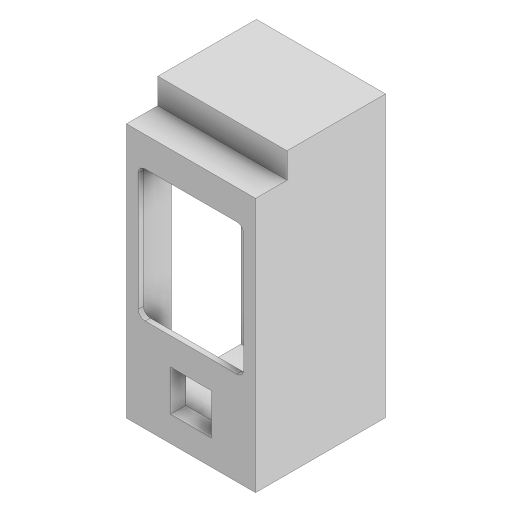
# Autodesk Inventor part: Part1
Saved by Autodesk Inventor 2023.3 (Build 273359000, 359)
## iProperties
Created: 2025-03-14
Part Number: Part1
Material: Generic
Document SubType Name: Modeling
Designer: David Zindović
Density: 1 g/cm^3
Appearance: Default
Author: David Zindović
Autodesk Inventor part; units mm, degrees
ref_plane "YZ Plane" through (0, 0, 0) normal (1, 0, 0) x (0, 1, 0)
ref_plane "XZ Plane" through (0, 0, 0) normal (0, 1, 0) x (-1, 0, 0)
ref_plane "XY Plane" through (0, 0, 0) normal (0, 0, 1) x (1, 0, 0)
sketch "Sketch1" plane through (0, 0, 0) normal (0, 0, 1) x (1, 0, 0)
  line L0 (-17, 22.5) -> (17, 22.5)
  line L1 (17, 22.5) -> (17, -22.5)
  line L2 (17, -22.5) -> (-17, -22.5)
  line L3 (-17, -22.5) -> (-17, 22.5)
  line L4 (-6, -25) -> (6, -25)
  line L5 (6, -25) -> (6, -37)
  line L6 (6, -37) -> (-6, -37)
  line L7 (-6, -37) -> (-6, -25)
  line L8 (-17, 28.5) -> (17, 28.5)
  line L9 (17, 28.5) -> (17, -29.5)
  line L10 (17, -29.5) -> (-17, -29.5)
  line L11 (-17, -29.5) -> (-17, 28.5)
  line L12 (-17, -29.5) -> (12, -29.5)
  line L13 (12, -29.5) -> (12, -42.5)
  line L14 (12, -42.5) -> (-17, -42.5)
  line L15 (-17, -42.5) -> (-17, -29.5)
  circle A0 centre (-14.5, -39.88) radius 1.5
  circle A1 centre (9.5, -39.88) radius 1.5
  circle A2 centre (-14.125, 25.5) radius 1.5
  circle A3 centre (14.125, 25.5) radius 1.5
  line L16 (-19, 30.5) -> (19, 30.5)
  line L17 (19, 30.5) -> (19, -44.5)
  line L18 (19, -44.5) -> (-19, -44.5)
  line L19 (-19, -44.5) -> (-19, 30.5)
  line L20 (12, -42.5) -> (17, -42.5)
  line L21 (17, -42.5) -> (17, -29.5)
  circle A4 centre (9.5, -39.88) radius 2.4
  circle A5 centre (-14.5, -39.88) radius 2.4
  circle A6 centre (14.125, 25.5) radius 2.4
  circle A7 centre (-14.125, 25.5) radius 2.4
  line L22 (-14.5, -36.7046) -> (-11.75, -38.2923)
  line L23 (-11.75, -38.2923) -> (-11.75, -41.4677)
  line L24 (-11.75, -41.4677) -> (-14.5, -43.0554)
  line L25 (-14.5, -43.0554) -> (-17.25, -41.4677)
  line L26 (-17.25, -41.4677) -> (-17.25, -38.2923)
  line L27 (-17.25, -38.2923) -> (-14.5, -36.7046)
  line L28 (-12.5373, 22.75) -> (-15.7127, 22.75)
  line L29 (-15.7127, 22.75) -> (-17.3004, 25.5)
  line L30 (-17.3004, 25.5) -> (-15.7127, 28.25)
  line L31 (-15.7127, 28.25) -> (-12.5373, 28.25)
  line L32 (-12.5373, 28.25) -> (-10.9496, 25.5)
  line L33 (-10.9496, 25.5) -> (-12.5373, 22.75)
  point P0 (0, 0)
  point P1 (0, 22.5)
  point P2 (17, 0)
  point P3 (0, -25)
  point P4 (0, -22.5)
  point P5 (0, 28.5)
  point P6 (-2.5, -42.5)
  point P7 (0, -44.5)
  point P8 (17, -22.5)
  dimension "d0" = 34
  dimension "d1" = 45
  dimension "d2" = 2.5
  dimension "d3" = 12
  dimension "d4" = 12
  dimension "d5" = 34
  dimension "d6" = 58
  dimension "d7" = 7
  dimension "d8" = 13
  dimension "d9" = 29
  dimension "d10" = 3
  dimension "d11" = 3
  dimension "d12" = 3
  dimension "d13" = 3
  dimension "d14" = 28.25
  dimension "d15" = 14.125
  dimension "d16" = 3
  dimension "d17" = 24
  dimension "d18" = 12
  dimension "d19" = 2.62
  dimension "d21" = 2
  dimension "d22" = 2
  dimension "d23" = 2
  dimension "d66" = 4.8
  dimension "d67" = 4.8
  dimension "d68" = 4.8
  dimension "d69" = 4.8
  dimension "d75" = 5.5
  dimension "d85" = 5.5
  constraints: 68 end point, 10 parallel, 8 centre point, 7 coincident, 7 midpoint, 6 horizontal, 5 perpendicular, 5 vertical alignment, 4 horizontal alignment, 1 collinear, 26 other
  measures "d0" distance of L0.start L0.end
  measures "d1" distance of L0.end L1.end
  measures "d2" distance between parallel lines of L2 L4
  measures "d3" distance of L5.end L6.end
  measures "d4" distance of L4.end L5.end
  measures "d5" distance of L8.start L8.end
  measures "d6" distance of L8.end L9.end
  measures "d7" distance between parallel lines of L2 L10
  measures "d8" distance of L12.end L13.end
  measures "d9" distance of L13.end L14.end
  measures "d10" diameter of A0
  measures "d11" diameter of A1
  measures "d12" diameter of A2
  measures "d13" diameter of A3
  measures "d14" distance of A3.centre A2.centre
  measures "d15" horizontal distance of point (0, 28.5) A3.centre
  measures "d16" distance from line of L8 A2.centre
  measures "d17" distance of A0.centre A1.centre
  measures "d18" horizontal distance of point (-2.5, -42.5) A1.centre
  measures "d19" distance from line of L14 A0.centre
  measures "d21" distance between parallel lines of L14 L18
  measures "d22" distance between parallel lines of L3 L19
  measures "d23" distance between parallel lines of L16 L8
  measures "d66" diameter of A4
  measures "d67" diameter of A5
  measures "d68" diameter of A6
  measures "d69" diameter of A7
  measures "d75" distance between parallel lines of L26 L23
  measures "d85" distance between parallel lines of L31 L28
extrude "Extrusion1" add sketch "Sketch1" along normal blind 4.5 contours L11 L29 L28 L33 L32 L31 L30 L8 L9 L0 | L2 L9 L10 L5 L4 L7 L11 | L29 L30 L11 | L11 L30 L31 L32 L33 L28 L29 | L10 L7 L6 L5 L13 L14 L24 L23 L22 L27 L15 | L21 L20 L13 L10 | L27 L22 L23 L24 L14 L25 L15 | L15 L25 L26 L27 | L25 L14 L15 | L14 L24 L25 | A0 | A1 | A2 | A3 | L16 L17 L18 L19 | A4 | A5 | A6 | A7
sketch "Sketch2" plane through (0, 0, 4.5) normal (0, 0, 1) x (1, 0, 0)
  line L0 (-17, -22.5) -> (-17, 22.5) projected
  line L1 (-17, 21.75) -> (17, 21.75)
  line L2 (17, 22.5) -> (17, -22.5) projected
  line L3 (-17, 22.5) -> (17, 22.5) projected
  line L4 (17, -22.5) -> (-17, -22.5) projected
  line L5 (-15.5, -22.5) -> (-15.5, 22.5)
  line L6 (-17, 22.5) -> (17, 22.5) projected
  line L7 (15.5, -22.5) -> (15.5, 22.5)
  line L8 (-17, -17) -> (17, -17)
  point P0 (0, 0)
  point P1 (-15.5, 21.75)
  point P2 (15.5, 21.75)
  point P3 (15.5, -17)
  point P4 (-15.5, -17)
  dimension "d26" = 0.75
  dimension "d27" = 1.5
  dimension "d28" = 1.5
  dimension "d29" = 5.5
  constraints: 8 end point, 8 point on line, 3 perpendicular, 1 horizontal
  measures "d26" distance between parallel lines of L3 L1
  measures "d27" distance between parallel lines of L0 L5
  measures "d28" distance between parallel lines of L2 L7
  measures "d29" distance between parallel lines of L8 L4
extrude "Extrusion2" add sketch "Sketch2" against normal blind 1.5 contours L0 L8 L5 L4 | L0 L1 L5 L8 | L5 L8 L7 L4 | L0 L3 L5 L1 | L7 L8 L2 L4 | L5 L3 L7 L1 | L7 L1 L2 L8 | L7 L3 L2 L1
fillet "Fillet1" radius 2 4 edges at (15.5, 21.75, 3.75) (-15.5, 21.75, 3.75) (-15.5, -17, 3.75) (15.5, -17, 3.75)
extrude "Extrusion3" add sketch "Sketch1" against normal blind 29.25 contours L29 L30 L11 | L15 L25 L26 L27 | L14 L24 L25 | L16 L17 L18 L19
sketch "Sketch3" plane through (-19, -44.5, 4.5) normal (-1, 0, 0) x (0, 0, 1)
  line L0 (-33.75, 2) -> (-33.75, 73) projected
  line L1 (-4.5, 2) -> (-33.75, 2) projected
  line L2 (-33.75, 73) -> (-11.25, 73)
  line L3 (-11.25, 73) -> (-11.25, 2)
  line L4 (-11.25, 2) -> (-33.75, 2)
  line L5 (-33.75, 2) -> (-33.75, 73)
  point P0 (-4.5, 44.5)
  dimension "d35" = 22.5
  constraints: 8 end point, 2 parallel, 1 horizontal, 1 perpendicular, 1 point on line
  measures "d35" distance of L3.end L4.end
extrude "Extrusion4" cut sketch "Sketch3" against normal up to surface (2 mm away)
sketch "Sketch4" plane through (0, 0, -29.25) normal (0, 0, -1) x (-1, 0, 0)
  line L0 (-19, 30.5) -> (-19, -44.5) projected
  line L1 (19, 30.5) -> (-19, 30.5) projected
  line L2 (-19, 30.5) -> (19, 30.5) projected
  line L3 (-19, 30.5) -> (19, 30.5)
  line L4 (19, 30.5) -> (19, -44.5)
  line L5 (19, -44.5) -> (-19, -44.5)
  line L6 (-19, -44.5) -> (-19, 30.5)
  point P0 (0, 0)
  constraints: 8 end point, 2 parallel, 1 horizontal, 1 perpendicular
extrude "Extrusion5" add sketch "Sketch4" along normal blind 2
sketch "Sketch5" plane through (-19, -44.5, 4.5) normal (-1, 0, 0) x (0, 0, 1)
  line L0 (-33.75, 73) -> (-11.25, 73) projected
  line L1 (-33.75, 73) -> (-11.25, 73)
  line L2 (-11.25, 73) -> (-11.25, 80.5)
  line L3 (-11.25, 80.5) -> (-33.75, 80.5)
  line L4 (-33.75, 80.5) -> (-33.75, 73)
  point P0 (-4.5, 44.5)
  dimension "d40" = 7.5
  constraints: 8 end point, 2 parallel, 1 horizontal, 1 perpendicular
  measures "d40" distance of L3.end L0.start
extrude "Extrusion6" cut sketch "Sketch5" against normal up to surface (36 mm away)
sketch "Sketch6" plane through (-19, -44.5, 4.5) normal (-1, 0, 0) x (0, 0, 1)
  line L0 (-33.75, 80.5) -> (-33.75, 73) projected
  line L1 (-11.25, 80.5) -> (-33.75, 80.5) projected
  line L2 (-11.25, 73) -> (-11.25, 80.5) projected
  line L3 (-35.75, 73) -> (-35.75, 82.5)
  line L4 (-35.75, 82.5) -> (-9.25, 82.5)
  line L5 (-9.25, 82.5) -> (-9.25, 73)
  line L6 (-35.75, 73) -> (-9.25, 73)
  line L7 (-4.5, 73) -> (-4.5, 67) projected
  point P0 (-4.5, 44.5)
  dimension "d43" = 2
  constraints: 8 end point, 1 perpendicular, 2 other
  measures "d43" distance between parallel lines of L1 L4
extrude "Extrusion7" add sketch "Sketch6" against normal up to surface (38 mm away) contours L0 L6 L3 L4 L5 L2 L1
sketch "Sketch7" plane through (19, -44.5, 4.5) normal (1, 0, 0) x (0, 0, -1)
  line L0 (11.25, 80.5) -> (11.25, 75) projected
  line L1 (33.75, 75) -> (11.25, 75) projected
  line L2 (33.75, 80.5) -> (11.25, 80.5) projected
  line L3 (33.75, 75) -> (33.75, 80.5) projected
  point P0 (4.5, 44.5)
extrude "Extrusion8" add sketch "Sketch7" against normal up to surface (2 mm away)
sketch "Sketch8" plane through (-17, -42.5, 0) normal (0, 1, 0) x (1, 0, 0)
  line L0 (34, 0) -> (34, 29.25) projected
  line L1 (-2, 29.25) -> (34, 29.25) projected
  line L2 (31.85, 29.25) -> (28.25, 29.25)
  line L3 (28.25, 29.25) -> (28.25, 20)
  line L4 (28.25, 20) -> (31.85, 20)
  line L5 (31.85, 20) -> (31.85, 29.25)
  point P0 (17, 0)
  dimension "d48" = 2.15
  dimension "d49" = 3.6
  dimension "d50" = 9.25
  constraints: 8 end point, 2 parallel, 1 horizontal, 1 perpendicular, 1 point on line
  measures "d48" distance between parallel lines of L0 L5
  measures "d49" distance of L3.end L4.end
  measures "d50" distance of L4.end L2.start
extrude "Extrusion9" cut sketch "Sketch8" against normal up to surface (2 mm away)
fillet "Fillet2" radius 0.75 4 edges at (14.85, -43.5, -29.25) (11.25, -43.5, -29.25) (11.25, -43.5, -20) (14.85, -43.5, -20)
sketch "Sketch9" plane through (17, -22.5, 3) normal (-1, 0, 0) x (0, 0, 1)
  circle A0 centre (-21.6, 19.25) radius 2.4
  line L0 (-9.75, -20) -> (-32.25, -20) projected
  line L1 (-32.25, -20) -> (-32.25, 58.5) projected
  circle A1 centre (-21.6, 19.25) radius 3.4
  point P0 (-3, 22.5)
  dimension "d54" = 4.8
  dimension "d55" = 39.25
  dimension "d56" = 10.65
  dimension "d57" = 1
  constraints: 2 centre point
  measures "d54" diameter of A0
  measures "d55" distance from line of L0 A0.centre
  measures "d56" distance from line of L1 A0.centre
  measures "d57" radial gap between concentric circles of A0 A1
extrude "Extrusion10" add sketch "Sketch9" along normal blind 3
chamfer "Chamfer1" distance 2 angle 45 1 edges at (17, -3.25, -22)
sketch "Sketch10" plane through (0, 0, -31.25) normal (0, 0, -1) x (-1, 0, 0)
  line L0 (12.6336, -38.0136) -> (16.3664, -38.0136) construction
  line L1 (16.3664, -38.0136) -> (16.3664, -41.7464) construction
  line L2 (16.3664, -41.7464) -> (12.6336, -41.7464) construction
  line L3 (12.6336, -41.7464) -> (12.6336, -38.0136) construction
  circle A0 centre (14.5, -39.88) radius 1.6
  circle A1 centre (14.125, 25.5) radius 1.6
  point P0 (0, 0)
  point P1 (14.5, -38.0136)
  point P2 (16.3664, -39.88)
  dimension "d64" = 3.7328
  dimension "d65" = 3.7328
  dimension "d95" = 3.2
  dimension "d96" = 3.2
  constraints: 8 end point, 2 centre point, 2 coincident, 2 midpoint, 2 parallel, 1 horizontal, 1 horizontal alignment, 1 perpendicular, 1 vertical alignment
  measures "d64" distance of L1.end L2.end
  measures "d65" distance of L0.end L1.end
  measures "d95" diameter of A0
  measures "d96" diameter of A1
extrude "Extrusion11" [suppressed]
sketch "Sketch11" plane through (-19, -44.5, 4.5) normal (0, -1, 0) x (1, 0, 0)
  line L0 (1.6, -3.7) -> (7.4, -3.7)
  line L1 (7.4, -3.7) -> (7.4, -1)
  line L2 (7.4, -1) -> (1.6, -1)
  line L3 (1.6, -1) -> (1.6, -3.7)
  line L4 (0, 0) -> (38, 0) projected
  point P0 (19, -4.5)
  point P1 (4.5, -4.5)
  point P2 (4.5, -3.7)
  dimension "d72" = 5.8
  dimension "d73" = 2.7
  dimension "d74" = 1
  constraints: 8 end point, 2 parallel, 1 horizontal, 1 midpoint, 1 perpendicular, 1 vertical alignment
  measures "d72" distance of L1.end L2.end
  measures "d73" distance of L2.end L0.start
  measures "d74" distance between parallel lines of L4 L2
extrude "Extrusion12" cut sketch "Sketch11" against normal up to surface (7.7954 mm away)
sketch "Sketch14" plane through (-19, -44.5, 4.5) normal (-1, 0, 0) x (0, 0, 1)
  line L0 (-3.7, 67.1) -> (-1, 67.1)
  line L1 (-1, 67.1) -> (-1, 72.9)
  line L2 (-1, 72.9) -> (-3.7, 72.9)
  line L3 (-3.7, 72.9) -> (-3.7, 67.1)
  line L4 (0, 75) -> (0, 0) projected
  point P0 (-4.5, 44.5)
  point P1 (-4.5, 70)
  point P2 (-3.7, 70)
  dimension "d86" = 5.8
  dimension "d87" = 2.7
  dimension "d88" = 1
  constraints: 8 end point, 2 parallel, 1 horizontal, 1 horizontal alignment, 1 midpoint, 1 perpendicular
  measures "d86" distance of L0.end L1.end
  measures "d87" distance of L0.start L0.end
  measures "d88" distance between parallel lines of L4 L1
extrude "Extrusion14" cut sketch "Sketch14" against normal up to surface (8.0504 mm away)
sketch "Sketch12" plane through (-11.6, -44.5, 3.5) normal (0, 0, -1) x (-1, 0, 0)
  line L0 (0, 0) -> (0, 7.7954) projected
  line L1 (5.8, 7.7954) -> (0, 7.7954) projected
  line L2 (5.8, 7.7954) -> (0, 7.7954) projected
  line L3 (0, 0) -> (0, 7.7954) projected
  line L4 (5.8, 0) -> (0, 0) projected
  line L5 (5.8, 0) -> (5.8, 7.7954) projected
  line L6 (2.9, 7.7954) -> (5.8, 6.1211)
  line L7 (5.65, 6.2077) -> (5.65, 3.0323)
  line L8 (5.65, 3.0323) -> (2.9, 1.4446)
  line L9 (2.9, 1.4446) -> (0.15, 3.0323)
  line L10 (0.15, 3.0323) -> (0.15, 6.2077)
  line L11 (0, 6.1211) -> (2.9, 7.7954)
  point P0 (-11.6, 44.5)
  point P1 (2.9, 4.62)
  dimension "d78" = 5.5
  constraints: 12 end point, 4 point on line, 2 midpoint, 2 vertical alignment, 13 other
  measures "d78" distance between parallel lines of L7 L10
extrude "Extrusion13" add sketch "Sketch12" along normal up to surface (2.7 mm away) contours L0 L1 L11 | L6 L1 L5
sketch "Sketch13" plane through (-19, 30.5, 4.5) normal (0, 1, 0) x (1, 0, 0)
  line L0 (7.775, 3.7) -> (1.975, 3.7)
  line L1 (1.975, 3.7) -> (1.975, 1)
  line L2 (1.975, 1) -> (7.775, 1)
  line L3 (7.775, 1) -> (7.775, 3.7)
  line L4 (38, 0) -> (0, 0) projected
  point P0 (19, 4.5)
  point P1 (7.775, 2.35)
  point P2 (1.975, 2.35)
  point P3 (4.875, 4.5)
  point P4 (4.875, 1)
  dimension "d81" = 5.8
  dimension "d82" = 2.7
  dimension "d83" = 1
  constraints: 8 end point, 3 midpoint, 2 parallel, 1 horizontal, 1 perpendicular, 1 vertical alignment
  measures "d81" distance of point (7.775, 2.35) point (1.975, 2.35)
  measures "d82" distance between parallel lines of L0 L2
  measures "d83" distance between parallel lines of L4 L2
sketch "Sketch15" plane through (-19, 22.6, 3.5) normal (0, 0, -1) x (-1, 0, 0)
  line L0 (-8.0504, 5.8) -> (-8.0504, 0) projected
  line L1 (0, 0) -> (-8.0504, 0) projected
  line L2 (0, 5.8) -> (0, 0) projected
  line L3 (0, 5.8) -> (-8.0504, 5.8) projected
  line L4 (-8.0504, 2.9) -> (-6.3761, 5.8)
  line L5 (-6.4627, 5.65) -> (-3.2873, 5.65)
  line L6 (-3.2873, 5.65) -> (-1.6996, 2.9)
  line L7 (-1.6996, 2.9) -> (-3.2873, 0.15)
  line L8 (-3.2873, 0.15) -> (-6.4627, 0.15)
  line L9 (-6.3761, 0) -> (-8.0504, 2.9)
  point P0 (-19, -22.6)
  point P1 (-4.875, 2.9)
  point P2 (-4.875, 2.9)
  constraints: 12 end point, 4 point on line, 1 coincident, 1 midpoint, 13 other
extrude "Extrusion15" add sketch "Sketch15" along normal up to surface (2.7 mm away) contours L3 L4 L0 | L9 L1 L0
extrude "Extrusion16" cut sketch "Sketch1" along normal up to surface (3.5 mm away) contours A0 | A2
extrude "Extrusion17" cut sketch "Sketch10" against normal up to surface (2 mm away)
sketch "Sketch16" plane through (0, 0, -31.25) normal (0, 0, -1) x (-1, 0, 0)
  circle A0 centre (14.125, 25.5) radius 1.6 projected
  circle A1 centre (14.5, -39.88) radius 1.6 projected
  line L0 (-19, 38) -> (-19, -44.5) projected
  line L1 (-19, -44.5) -> (19, -44.5) projected
  line L2 (19, -44.5) -> (19, 38) projected
  line L3 (19, 38) -> (-19, 38) projected
  circle A2 centre (14.5, -39.88) radius 3.2
  circle A3 centre (14.125, 25.5) radius 1.6 projected
  circle A4 centre (14.125, 25.5) radius 3.2
  line L4 (0.0016, 10.5085) -> (0.8575, 11.52)
  line L5 (0.8575, 11.52) -> (1.8695, 12.3963)
  line L6 (1.8695, 12.3963) -> (5.466, 15.2223)
  line L7 (5.466, 15.2223) -> (7.072, 16.8394)
  line L8 (7.072, 16.8394) -> (7.7025, 17.7676)
  line L9 (7.7025, 17.7676) -> (8.1706, 18.8013)
  line L10 (8.1706, 18.8013) -> (8.4174, 19.8205)
  line L11 (8.4174, 19.8205) -> (8.5056, 20.9394)
  line L12 (8.5056, 20.9394) -> (8.4166, 22.0551)
  line L13 (8.4166, 22.0551) -> (8.1325, 23.0653)
  line L14 (8.1325, 23.0653) -> (7.7393, 23.7945)
  line L15 (7.7393, 23.7945) -> (7.2255, 24.4195)
  line L16 (7.2255, 24.4195) -> (5.9179, 25.3288)
  line L17 (5.9179, 25.3288) -> (4.3738, 25.7336)
  line L18 (4.3738, 25.7336) -> (3.5639, 25.7286)
  line L19 (3.5639, 25.7286) -> (2.7567, 25.5754)
  line L20 (2.7567, 25.5754) -> (1.5044, 24.9629)
  line L21 (1.5044, 24.9629) -> (0.5395, 23.9554)
  line L22 (0.5395, 23.9554) -> (0.2453, 23.3728)
  line L23 (0.2453, 23.3728) -> (-0.0924, 22.8314)
  line L24 (-0.0924, 22.8314) -> (-0.3516, 23.6617)
  line L25 (-0.3516, 23.6617) -> (-0.8594, 24.3774)
  line L26 (-0.8594, 24.3774) -> (-1.5428, 25.0076)
  line L27 (-1.5428, 25.0076) -> (-2.3262, 25.4447)
  line L28 (-2.3262, 25.4447) -> (-3.1769, 25.6945)
  line L29 (-3.1769, 25.6945) -> (-4.0616, 25.7625)
  line L30 (-4.0616, 25.7625) -> (-4.9472, 25.6543)
  line L31 (-4.9472, 25.6543) -> (-5.8007, 25.3757)
  line L32 (-5.8007, 25.3757) -> (-6.5892, 24.9325)
  line L33 (-6.5892, 24.9325) -> (-7.2795, 24.3303)
  line L34 (-7.2795, 24.3303) -> (-8.1248, 23.0283)
  line L35 (-8.1248, 23.0283) -> (-8.4534, 21.5194)
  line L36 (-8.4534, 21.5194) -> (-8.4172, 20.0499)
  line L37 (-8.4172, 20.0499) -> (-8.0923, 18.6142)
  line L38 (-8.0923, 18.6142) -> (-7.6666, 17.6967)
  line L39 (-7.6666, 17.6967) -> (-7.1065, 16.8648)
  line L40 (-7.1065, 16.8648) -> (-5.6938, 15.4035)
  line L41 (-5.6938, 15.4035) -> (-2.4733, 12.9074)
  line L42 (-2.4733, 12.9074) -> (-0.8525, 11.4885)
  line L43 (-0.8525, 11.4885) -> (-0.4527, 10.9583)
  line L44 (-0.4527, 10.9583) -> (0.0016, 10.5085)
  line L45 (-0.0767, -10.1601) -> (0.7792, -9.1486)
  line L46 (0.7792, -9.1486) -> (1.7912, -8.2723)
  line L47 (1.7912, -8.2723) -> (5.3877, -5.4463)
  line L48 (5.3877, -5.4463) -> (6.9937, -3.8292)
  line L49 (6.9937, -3.8292) -> (7.6242, -2.901)
  line L50 (7.6242, -2.901) -> (8.0923, -1.8673)
  line L51 (8.0923, -1.8673) -> (8.3392, -0.8481)
  line L52 (8.3392, -0.8481) -> (8.4273, 0.2708)
  line L53 (8.4273, 0.2708) -> (8.3384, 1.3866)
  line L54 (8.3384, 1.3866) -> (8.0542, 2.3968)
  line L55 (8.0542, 2.3968) -> (7.661, 3.1259)
  line L56 (7.661, 3.1259) -> (7.1472, 3.7509)
  line L57 (7.1472, 3.7509) -> (5.8396, 4.6603)
  line L58 (5.8396, 4.6603) -> (4.2955, 5.0651)
  line L59 (4.2955, 5.0651) -> (3.4856, 5.0601)
  line L60 (3.4856, 5.0601) -> (2.6784, 4.9069)
  line L61 (2.6784, 4.9069) -> (1.4261, 4.2943)
  line L62 (1.4261, 4.2943) -> (0.4612, 3.2868)
  line L63 (0.4612, 3.2868) -> (0.167, 2.7042)
  line L64 (0.167, 2.7042) -> (-0.1706, 2.1629)
  line L65 (-0.1706, 2.1629) -> (-0.4299, 2.9931)
  line L66 (-0.4299, 2.9931) -> (-0.9377, 3.7088)
  line L67 (-0.9377, 3.7088) -> (-1.6211, 4.3391)
  line L68 (-1.6211, 4.3391) -> (-2.4045, 4.7761)
  line L69 (-2.4045, 4.7761) -> (-3.2552, 5.0259)
  line L70 (-3.2552, 5.0259) -> (-4.1399, 5.0939)
  line L71 (-4.1399, 5.0939) -> (-5.0255, 4.9857)
  line L72 (-5.0255, 4.9857) -> (-5.879, 4.7071)
  line L73 (-5.879, 4.7071) -> (-6.6675, 4.2639)
  line L74 (-6.6675, 4.2639) -> (-7.3578, 3.6617)
  line L75 (-7.3578, 3.6617) -> (-8.2031, 2.3597)
  line L76 (-8.2031, 2.3597) -> (-8.5317, 0.8508)
  line L77 (-8.5317, 0.8508) -> (-8.4955, -0.6187)
  line L78 (-8.4955, -0.6187) -> (-8.1706, -2.0543)
  line L79 (-8.1706, -2.0543) -> (-7.7449, -2.9719)
  line L80 (-7.7449, -2.9719) -> (-7.1847, -3.8038)
  line L81 (-7.1847, -3.8038) -> (-5.7721, -5.2651)
  line L82 (-5.7721, -5.2651) -> (-2.5516, -7.7611)
  line L83 (-2.5516, -7.7611) -> (-0.9308, -9.1801)
  line L84 (-0.9308, -9.1801) -> (-0.531, -9.7103)
  line L85 (-0.531, -9.7103) -> (-0.0767, -10.1601)
  line L86 (0.0016, -31.7681) -> (0.8575, -30.7566)
  line L87 (0.8575, -30.7566) -> (1.8695, -29.8803)
  line L88 (1.8695, -29.8803) -> (5.466, -27.0543)
  line L89 (5.466, -27.0543) -> (7.072, -25.4372)
  line L90 (7.072, -25.4372) -> (7.7025, -24.509)
  line L91 (7.7025, -24.509) -> (8.1706, -23.4753)
  line L92 (8.1706, -23.4753) -> (8.4174, -22.4561)
  line L93 (8.4174, -22.4561) -> (8.5056, -21.3372)
  line L94 (8.5056, -21.3372) -> (8.4166, -20.2215)
  line L95 (8.4166, -20.2215) -> (8.1325, -19.2113)
  line L96 (8.1325, -19.2113) -> (7.7393, -18.4821)
  line L97 (7.7393, -18.4821) -> (7.2255, -17.8572)
  line L98 (7.2255, -17.8572) -> (5.9179, -16.9478)
  line L99 (5.9179, -16.9478) -> (4.3738, -16.543)
  line L100 (4.3738, -16.543) -> (3.5639, -16.548)
  line L101 (3.5639, -16.548) -> (2.7567, -16.7012)
  line L102 (2.7567, -16.7012) -> (1.5044, -17.3137)
  line L103 (1.5044, -17.3137) -> (0.5395, -18.3212)
  line L104 (0.5395, -18.3212) -> (0.2453, -18.9038)
  line L105 (0.2453, -18.9038) -> (-0.0924, -19.4452)
  line L106 (-0.0924, -19.4452) -> (-0.3516, -18.6149)
  line L107 (-0.3516, -18.6149) -> (-0.8594, -17.8992)
  line L108 (-0.8594, -17.8992) -> (-1.5428, -17.269)
  line L109 (-1.5428, -17.269) -> (-2.3262, -16.8319)
  line L110 (-2.3262, -16.8319) -> (-3.1769, -16.5821)
  line L111 (-3.1769, -16.5821) -> (-4.0616, -16.5141)
  line L112 (-4.0616, -16.5141) -> (-4.9472, -16.6223)
  line L113 (-4.9472, -16.6223) -> (-5.8007, -16.9009)
  line L114 (-5.8007, -16.9009) -> (-6.5892, -17.3441)
  line L115 (-6.5892, -17.3441) -> (-7.2795, -17.9463)
  line L116 (-7.2795, -17.9463) -> (-8.1248, -19.2483)
  line L117 (-8.1248, -19.2483) -> (-8.4534, -20.7572)
  line L118 (-8.4534, -20.7572) -> (-8.4172, -22.2267)
  line L119 (-8.4172, -22.2267) -> (-8.0923, -23.6624)
  line L120 (-8.0923, -23.6624) -> (-7.6666, -24.5799)
  line L121 (-7.6666, -24.5799) -> (-7.1065, -25.4118)
  line L122 (-7.1065, -25.4118) -> (-5.6938, -26.8731)
  line L123 (-5.6938, -26.8731) -> (-2.4733, -29.3692)
  line L124 (-2.4733, -29.3692) -> (-0.8525, -30.7881)
  line L125 (-0.8525, -30.7881) -> (-0.4527, -31.3184)
  line L126 (-0.4527, -31.3184) -> (0.0016, -31.7681)
  point P0 (0, 0)
  point P1 (0.5395, -18.3212)
  point P2 (-0.9308, -9.1801)
  point P3 (-0.8525, 11.4885)
  point P4 (0.8575, 11.52)
  dimension "d99" = 6.4
  dimension "d100" = 6.4
  constraints: 246 end point, 2 centre point, 2 coincident
  measures "d99" diameter of A2
  measures "d100" diameter of A4
extrude "Extrusion18" add sketch "Sketch16" along normal blind 2.5 contours L3 L2 L1 L0
sketch "Sketch17" plane through (0, 0, -31.25) normal (0, 0, -1) x (-1, 0, 0)
  line L0 (0.0016, 10.5085) -> (0.8575, 11.52) projected
  line L1 (0.8575, 11.52) -> (1.8695, 12.3963) projected
  line L2 (1.8695, 12.3963) -> (5.466, 15.2223) projected
  line L3 (5.466, 15.2223) -> (7.072, 16.8394) projected
  line L4 (7.072, 16.8394) -> (7.7025, 17.7676) projected
  line L5 (7.7025, 17.7676) -> (8.1706, 18.8013) projected
  line L6 (8.1706, 18.8013) -> (8.4174, 19.8205) projected
  line L7 (8.4174, 19.8205) -> (8.5056, 20.9394) projected
  line L8 (8.5056, 20.9394) -> (8.4166, 22.0551) projected
  line L9 (8.4166, 22.0551) -> (8.1325, 23.0653) projected
  line L10 (8.1325, 23.0653) -> (7.7393, 23.7945) projected
  line L11 (7.7393, 23.7945) -> (7.2255, 24.4195) projected
  line L12 (7.2255, 24.4195) -> (5.9179, 25.3288) projected
  line L13 (5.9179, 25.3288) -> (4.3738, 25.7336) projected
  line L14 (4.3738, 25.7336) -> (3.5639, 25.7286) projected
  line L15 (3.5639, 25.7286) -> (2.7567, 25.5754) projected
  line L16 (2.7567, 25.5754) -> (1.5044, 24.9629) projected
  line L17 (1.5044, 24.9629) -> (0.5395, 23.9554) projected
  line L18 (0.5395, 23.9554) -> (0.2453, 23.3728) projected
  line L19 (0.2453, 23.3728) -> (-0.0924, 22.8314) projected
  line L20 (-0.0924, 22.8314) -> (-0.3516, 23.6617) projected
  line L21 (-0.3516, 23.6617) -> (-0.8594, 24.3774) projected
  line L22 (-0.8594, 24.3774) -> (-1.5428, 25.0076) projected
  line L23 (-1.5428, 25.0076) -> (-2.3262, 25.4447) projected
  line L24 (-2.3262, 25.4447) -> (-3.1769, 25.6945) projected
  line L25 (-3.1769, 25.6945) -> (-4.0616, 25.7625) projected
  line L26 (-4.0616, 25.7625) -> (-4.9472, 25.6543) projected
  line L27 (-4.9472, 25.6543) -> (-5.8007, 25.3757) projected
  line L28 (-5.8007, 25.3757) -> (-6.5892, 24.9325) projected
  line L29 (-6.5892, 24.9325) -> (-7.2795, 24.3303) projected
  line L30 (-7.2795, 24.3303) -> (-8.1248, 23.0283) projected
  line L31 (-8.1248, 23.0283) -> (-8.4534, 21.5194) projected
  line L32 (-8.4534, 21.5194) -> (-8.4172, 20.0499) projected
  line L33 (-8.4172, 20.0499) -> (-8.0923, 18.6142) projected
  line L34 (-8.0923, 18.6142) -> (-7.6666, 17.6967) projected
  line L35 (-7.6666, 17.6967) -> (-7.1065, 16.8648) projected
  line L36 (-7.1065, 16.8648) -> (-5.6938, 15.4035) projected
  line L37 (-5.6938, 15.4035) -> (-2.4733, 12.9074) projected
  line L38 (-2.4733, 12.9074) -> (-0.8525, 11.4885) projected
  line L39 (-0.8525, 11.4885) -> (-0.4527, 10.9583) projected
  line L40 (-0.4527, 10.9583) -> (0.0016, 10.5085) projected
  line L41 (1.7912, -8.2723) -> (5.3877, -5.4463) projected
  line L42 (5.3877, -5.4463) -> (6.9937, -3.8292) projected
  line L43 (6.9937, -3.8292) -> (7.6242, -2.901) projected
  line L44 (7.6242, -2.901) -> (8.0923, -1.8673) projected
  line L45 (8.0923, -1.8673) -> (8.3392, -0.8481) projected
  line L46 (8.3392, -0.8481) -> (8.4273, 0.2708) projected
  line L47 (8.4273, 0.2708) -> (8.3384, 1.3866) projected
  line L48 (8.3384, 1.3866) -> (8.0542, 2.3968) projected
  line L49 (8.0542, 2.3968) -> (7.661, 3.1259) projected
  line L50 (7.661, 3.1259) -> (7.1472, 3.7509) projected
  line L51 (7.1472, 3.7509) -> (5.8396, 4.6603) projected
  line L52 (5.8396, 4.6603) -> (4.2955, 5.0651) projected
  line L53 (4.2955, 5.0651) -> (3.4856, 5.0601) projected
  line L54 (3.4856, 5.0601) -> (2.6784, 4.9069) projected
  line L55 (2.6784, 4.9069) -> (1.4261, 4.2943) projected
  line L56 (1.4261, 4.2943) -> (0.4612, 3.2868) projected
  line L57 (0.4612, 3.2868) -> (0.167, 2.7042) projected
  line L58 (0.167, 2.7042) -> (-0.1706, 2.1629) projected
  line L59 (-0.1706, 2.1629) -> (-0.4299, 2.9931) projected
  line L60 (-0.4299, 2.9931) -> (-0.9377, 3.7088) projected
  line L61 (-0.9377, 3.7088) -> (-1.6211, 4.3391) projected
  line L62 (-1.6211, 4.3391) -> (-2.4045, 4.7761) projected
  line L63 (-2.4045, 4.7761) -> (-3.2552, 5.0259) projected
  line L64 (-3.2552, 5.0259) -> (-4.1399, 5.0939) projected
  line L65 (-4.1399, 5.0939) -> (-5.0255, 4.9857) projected
  line L66 (-5.0255, 4.9857) -> (-5.879, 4.7071) projected
  line L67 (-5.879, 4.7071) -> (-6.6675, 4.2639) projected
  line L68 (-6.6675, 4.2639) -> (-7.3578, 3.6617) projected
  line L69 (-7.3578, 3.6617) -> (-8.2031, 2.3597) projected
  line L70 (-8.2031, 2.3597) -> (-8.5317, 0.8508) projected
  line L71 (-8.5317, 0.8508) -> (-8.4955, -0.6187) projected
  line L72 (-8.4955, -0.6187) -> (-8.1706, -2.0543) projected
  line L73 (-8.1706, -2.0543) -> (-7.7449, -2.9719) projected
  line L74 (-7.7449, -2.9719) -> (-7.1847, -3.8038) projected
  line L75 (-7.1847, -3.8038) -> (-5.7721, -5.2651) projected
  line L76 (-5.7721, -5.2651) -> (-2.5516, -7.7611) projected
  line L77 (-2.5516, -7.7611) -> (-0.9308, -9.1801) projected
  line L78 (-0.9308, -9.1801) -> (-0.531, -9.7103) projected
  line L79 (-0.531, -9.7103) -> (-0.0767, -10.1601) projected
  line L80 (-0.0767, -10.1601) -> (0.7792, -9.1486) projected
  line L81 (0.7792, -9.1486) -> (1.7912, -8.2723) projected
  line L82 (1.8695, -29.8803) -> (5.466, -27.0543) projected
  line L83 (5.466, -27.0543) -> (7.072, -25.4372) projected
  line L84 (7.072, -25.4372) -> (7.7025, -24.509) projected
  line L85 (7.7025, -24.509) -> (8.1706, -23.4753) projected
  line L86 (8.1706, -23.4753) -> (8.4174, -22.4561) projected
  line L87 (8.4174, -22.4561) -> (8.5056, -21.3372) projected
  line L88 (8.5056, -21.3372) -> (8.4166, -20.2215) projected
  line L89 (8.4166, -20.2215) -> (8.1325, -19.2113) projected
  line L90 (8.1325, -19.2113) -> (7.7393, -18.4821) projected
  line L91 (7.7393, -18.4821) -> (7.2255, -17.8572) projected
  line L92 (7.2255, -17.8572) -> (5.9179, -16.9478) projected
  line L93 (5.9179, -16.9478) -> (4.3738, -16.543) projected
  line L94 (4.3738, -16.543) -> (3.5639, -16.548) projected
  line L95 (3.5639, -16.548) -> (2.7567, -16.7012) projected
  line L96 (2.7567, -16.7012) -> (1.5044, -17.3137) projected
  line L97 (1.5044, -17.3137) -> (0.5395, -18.3212) projected
  line L98 (0.5395, -18.3212) -> (0.2453, -18.9038) projected
  line L99 (0.2453, -18.9038) -> (-0.0924, -19.4452) projected
  line L100 (-0.0924, -19.4452) -> (-0.3516, -18.6149) projected
  line L101 (-0.3516, -18.6149) -> (-0.8594, -17.8992) projected
  line L102 (-0.8594, -17.8992) -> (-1.5428, -17.269) projected
  line L103 (-1.5428, -17.269) -> (-2.3262, -16.8319) projected
  line L104 (-2.3262, -16.8319) -> (-3.1769, -16.5821) projected
  line L105 (-3.1769, -16.5821) -> (-4.0616, -16.5141) projected
  line L106 (-4.0616, -16.5141) -> (-4.9472, -16.6223) projected
  line L107 (-4.9472, -16.6223) -> (-5.8007, -16.9009) projected
  line L108 (-5.8007, -16.9009) -> (-6.5892, -17.3441) projected
  line L109 (-6.5892, -17.3441) -> (-7.2795, -17.9463) projected
  line L110 (-7.2795, -17.9463) -> (-8.1248, -19.2483) projected
  line L111 (-8.1248, -19.2483) -> (-8.4534, -20.7572) projected
  line L112 (-8.4534, -20.7572) -> (-8.4172, -22.2267) projected
  line L113 (-8.4172, -22.2267) -> (-8.0923, -23.6624) projected
  line L114 (-8.0923, -23.6624) -> (-7.6666, -24.5799) projected
  line L115 (-7.6666, -24.5799) -> (-7.1065, -25.4118) projected
  line L116 (-7.1065, -25.4118) -> (-5.6938, -26.8731) projected
  line L117 (-5.6938, -26.8731) -> (-2.4733, -29.3692) projected
  line L118 (-2.4733, -29.3692) -> (-0.8525, -30.7881) projected
  line L119 (-0.8525, -30.7881) -> (-0.4527, -31.3184) projected
  line L120 (-0.4527, -31.3184) -> (0.0016, -31.7681) projected
  line L121 (0.0016, -31.7681) -> (0.8575, -30.7566) projected
  line L122 (0.8575, -30.7566) -> (1.8695, -29.8803) projected
  point P0 (0, 0)
extrude "Extrusion19" add sketch "Sketch17" along normal blind 1.5
equation "\"d15\" = 0.5 * d14"
equation "\"d18\" = 0.5 * d17"
equation "\"d23\" = d21"
equation "\"d28\" = d27"
equation "\"d65\" = d64"
equation "\"d96\" = d95"
equation "\"d100\" = d99"
body "Solid1"
